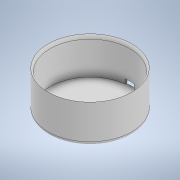
# Autodesk Inventor part: Tapa motor775
Saved by Autodesk Inventor 2021 (Build 250183000, 183)
## iProperties
Created: 2022-10-08
Part Number: Tapa motor775
Material: Genérico
Document SubType Name: Modeling
Designer: sergi
Density: 1 g/cm^3
Appearance: Valor por defecto
Author: sergi
Autodesk Inventor part; units mm, degrees
ref_plane "YZ Plane" through (0, 0, 0) normal (1, 0, 0) x (0, 1, 0)
ref_plane "XZ Plane" through (0, 0, 0) normal (0, 1, 0) x (-1, 0, 0)
ref_plane "XY Plane" through (0, 0, 0) normal (0, 0, 1) x (1, 0, 0)
sketch "Boceto1" plane through (0, 0, 0) normal (0, 1, 0) x (-1, 0, 0)
  circle A0 centre (0, 0) radius 22
  dimension "d0" = 44
  constraints: 1 centre point, 1 coincident
  measures "d0" diameter of A0
extrude "Extrusión1" add sketch "Boceto1" along normal blind 20
shell "Vaciado1" thickness 1 removed faces 1 at (6.4933, 20, -3.408)
sketch "Boceto3" plane through (0, 1, 0) normal (0, 1, 0) x (1, 0, 0)
  circle A0 centre (0, 0) radius 21 projected
  line L0 (2.4, 19.75) -> (-2.4, 19.75)
  line L1 (-2.4, 19.75) -> (-2.4, 22.25)
  line L2 (-2.4, 22.25) -> (2.4, 22.25)
  line L3 (2.4, 22.25) -> (2.4, 19.75)
  line L4 (2.4, 19.75) -> (-2.4, 22.25) construction
  line L5 (-2.4, 19.75) -> (2.4, 22.25) construction
  point P0 (0, 21)
  dimension "d4" = 4.8
  dimension "d5" = 2.5
  constraints: 12 end point, 2 midpoint, 2 parallel, 1 horizontal, 1 perpendicular, 1 vertical alignment, 1 other
  measures "d4" distance of L1.end L2.end
  measures "d5" distance of L0.end L1.end
extrude "Extrusión2" cut sketch "Boceto3" along normal blind 2.5 contours L3 L0 L1 A0 | A0 L1 L2 L3 picked at (-0.2672, 20.1616)
fillet "Empalme1" radius 2 2 edges at (22, 0, 0) (21, 20, 0)
